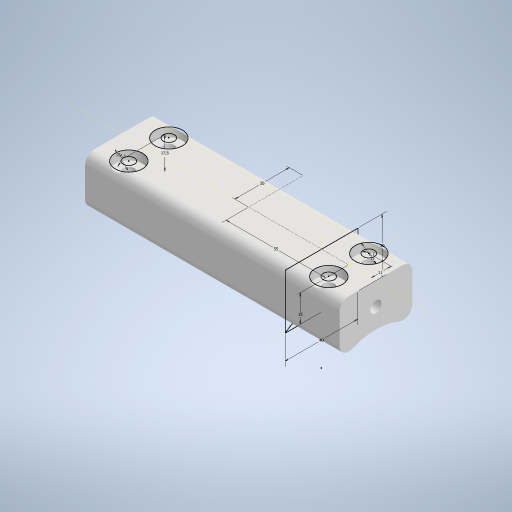
# Autodesk Inventor part: uMule-ogranicznik_koła
Saved by Autodesk Inventor 2024.2 (Build 282272000, 272)
## iProperties
Created: 2024-10-21
Part Number: uMule-ogranicznik_koła
Material: Ogólny
Document SubType Name: Modeling
Designer: owozn
Density: 1 g/cm^3
Appearance: Domyślna
Author: owozn
Autodesk Inventor part; units mm, degrees
ref_plane "YZ Plane" through (0, 0, 0) normal (1, 0, 0) x (0, 1, 0)
ref_plane "XZ Plane" through (0, 0, 0) normal (0, 1, 0) x (-1, 0, 0)
ref_plane "XY Plane" through (0, 0, 0) normal (0, 0, 1) x (1, 0, 0)
sketch "Szkic1" plane through (0, 0, 0) normal (0, 1, 0) x (-1, 0, 0)
  line L0 (15, 20) -> (-15, 20)
  line L1 (-15, 20) -> (-15, -20)
  line L2 (-15, -20) -> (15, -20)
  line L3 (15, -20) -> (15, 20)
  line L4 (15, 20) -> (-15, -20) construction
  line L5 (-15, 20) -> (15, -20) construction
  line L6 (0, -28) -> (0, 28) construction
  line L7 (21, 0) -> (-21, 0) construction
  point P0 (0, 0)
  dimension "d0" = 30
  dimension "d1" = 40
  constraints: 12 end point, 2 midpoint, 2 parallel, 1 horizontal, 1 perpendicular
  measures "d0" distance of L2.end L1.end
  measures "d1" distance of L1.end L0.end
extrude "Wyciągnięcie proste1" add sketch "Szkic1" along normal blind 30
sketch "Szkic2" plane through (-15, 0, -20) normal (-1, 0, 0) x (0, 0, 1)
  line L0 (-8, 0) -> (48, 0) construction
  line L1 (20, -6) -> (20, 36) construction
  line L2 (40, 30) -> (0, 30)
  line L3 (0, 30) -> (0, 0)
  line L4 (0, 0) -> (40, 0)
  line L5 (40, 0) -> (40, 30)
  line L6 (40, 30) -> (0, 0) construction
  line L7 (0, 30) -> (40, 0) construction
  line L8 (0, 0) -> (40, 0) projected
  arc A0 (40, 0) -> (0, 0) centre (20, -26.6667) ccw
  point P0 (20, 0)
  point P1 (20, 15)
  point P2 (20, 0)
  point P3 (0, 0)
  point P4 (0, 0)
  dimension "d4" = 40
  dimension "d5" = 30
  dimension "d6" = 15
  constraints: 12 end point, 4 midpoint, 2 parallel, 2 point on circle, 1 centre point, 1 horizontal, 1 perpendicular, 1 tangent
  measures "d4" distance of L4.end L3.end
  measures "d5" distance of L3.end L2.end
  measures "d6" distance of point (20, 0) point (20, 15)
extrude "Wyciągnięcie proste2" add sketch "Szkic2" along normal blind 110 contours L5 A0 L3 L2
extrude "Wyciągnięcie proste3" cut sketch "Szkic2" along normal through all both and the other way through all contours L4 A0
fillet "Zaokrąglenie1" radius 5 6 edges at (0, 0, 20) (-70, 0, 20) (0, 0, -20) (-70, 0, -20) (-55, 30, 20) (-55, 30, -20)
sketch "Szkic3" plane through (0, 30, 0) normal (0, 1, 0) x (1, 0, 0)
  line L0 (-153, 0) -> (43, 0) construction
  line L1 (0, 28) -> (0, -28) construction
  circle A0 centre (0, 11) radius 7.5
  circle A1 centre (0, 11) radius 3.05
  circle A2 centre (0, -11) radius 7.5
  circle A3 centre (0, -11) radius 3.05
  line L2 (0, 0) -> (-55, 0) construction
  line L3 (-125, 15) -> (15, 15) construction
  line L4 (-55, 0) -> (-55, 30) construction
  circle A4 centre (-110, 11) radius 7.5
  circle A5 centre (-110, 11) radius 3.05
  circle A6 centre (-110, -11) radius 7.5
  circle A7 centre (-110, -11) radius 3.05
  dimension "d12" = 15
  dimension "d13" = 6.1
  dimension "d14" = 11
  dimension "d21" = 55
  dimension "d23" = 30
  constraints: 8 centre point, 6 symmetric about line, 4 coincident, 4 end point, 1 midpoint, 1 point on line, 1 vertical, 6 other
  measures "d12" diameter of A0
  measures "d13" diameter of A1
  measures "d14" distance from line of L0 A0.centre
  measures "d21" distance of L2.start L2.end
  measures "d23" distance of L2.end L4.end
extrude "Wyciągnięcie proste4" cut sketch "Szkic3" against normal through all contours A0 | A1 | A2 | A3 | A4 | A5 | A6 | A7
extrude "Wyciągnięcie proste5" add sketch "Szkic3" against normal blind 23.5
extrude "Wyciągnięcie proste6" cut sketch "Szkic3" against normal blind 5
sketch "Szkic5" plane through (0, 30, 0) normal (0, 1, 0) x (1, 0, 0)
  point P0 (0, 0)
sketch "Szkic6" plane through (-125, 0, -20) normal (-1, 0, 0) x (0, 0, 1)
  line L0 (-8, 0) -> (48, 0) construction
  line L1 (20, -6.0006) -> (20, 36.0033) construction
  circle A0 centre (20, 17.5) radius 7.5
  circle A1 centre (20, 17.5) radius 3.05
  point P0 (20, 0)
  dimension "d24" = 15
  dimension "d25" = 6.1
  dimension "d26" = 17.5
  constraints: 2 centre point, 1 coincident, 1 point on line
  measures "d24" diameter of A0
  measures "d25" diameter of A1
  measures "d26" distance from line of L0 A0.centre
extrude "Wyciągnięcie proste7" cut sketch "Szkic6" against normal through all contours A1
hole "Otwór1" at (-110, 30, 11) at (-110, 30, -11) at (0, 30, 11) at (0, 30, -11) direction (0, -1, 0) diameter 6.2 end through all
